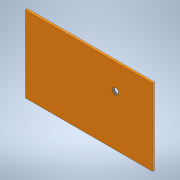
# Autodesk Inventor part: KaptonReedNozzleSheet
Saved by Autodesk Inventor 2021 (Build 250183000, 183)
## iProperties
Created: 2022-02-03
Part Number: KaptonReedNozzleSheet
Material: Generic
Document SubType Name: Sheet Metal
Designer: Unit-005
Density: 1 g/cm^3
Sheet Metal Rule: Default
Appearance: Default
Author: Unit-005
Autodesk Inventor part; units mm, degrees
ref_plane "YZ Plane" through (0, 0, 0) normal (1, 0, 0) x (0, 1, 0)
ref_plane "XZ Plane" through (0, 0, 0) normal (0, 1, 0) x (-1, 0, 0)
ref_plane "XY Plane" through (0, 0, 0) normal (0, 0, 1) x (1, 0, 0)
sketch "Sketch1" plane through (0, 0, 0) normal (0, 0, 1) x (1, 0, 0)
  line L0 (3.175, 1.27) -> (3.175, -2.54)
  line L1 (3.175, -2.54) -> (-3.175, -2.54)
  line L2 (-3.175, -2.54) -> (-3.175, 1.27)
  line L3 (-4.445, 0) -> (4.445, 0) projected
  line L4 (3.175, 1.27) -> (-3.175, 1.27)
  line L5 (0, -3.302) -> (0, 2.032) projected
  point P0 (0, 0)
  dimension "d0" = 6.35
  dimension "d12" = 2.54
  dimension "d14" = 1.27
  constraints: 8 end point, 1 parallel, 1 perpendicular, 1 other
  measures "d0" distance of L0.end L1.end
  measures "d12" distance between parallel lines of L3 L1
  measures "d14" distance between parallel lines of L4 L3
extrude "Extrusion1" add sketch "Sketch1" along normal blind 0.1016
sketch "Sketch2" plane through (0, 0, 0.1016) normal (0, 0, 1) x (1, 0, 0)
  line L0 (-4.445, 0) -> (4.445, 0) projected
  line L1 (0, -3.302) -> (0, 2.032) projected
  line L2 (-3.175, -2.54) -> (3.175, -2.54) projected
  line L3 (3.175, -2.54) -> (3.175, 1.27) projected
  line L4 (-3.175, 1.27) -> (-3.175, -2.54) projected
  circle A0 centre (1.325, 0) radius 0.1524
  line L5 (3.175, 1.27) -> (-3.175, 1.27) projected
  point P0 (0, 0)
  dimension "d4" = 0.3048
  dimension "d5" = 1.85
  constraints: 1 centre point, 1 point on line
  measures "d4" diameter of A0
  measures "d5" distance from line of L3 A0.centre
extrude "Extrusion2" cut sketch "Sketch2" against normal through all contours A0 L0 | L0 A0
pattern_linear "Rectangular Pattern1" [suppressed]
equation "\"BendRadius\" = Thickness"
equation "\"BendReliefWidth\" = Thickness"
equation "\"BendReliefDepth\" = 0.5 * Thickness"
equation "\"CornerReliefSize\" = 4 * Thickness"
equation "\"MinimumRemnant\" = 2 * Thickness"
equation "\"TransitionRadius\" = BendRadius"
equation "\"JacobiRadiusSize\" = BendRadius"
equation "\"GapSize\" = Thickness"
equation "\"Thickness\" = 3.048"
body "Solid1"
